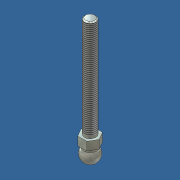
# Autodesk Inventor part: 21.1846 THREADED STUD 10mm
Saved by Autodesk Inventor 2016 (Build 200138000, 138)
## iProperties
Created: 2007-03-28
Part Number: 21.1846 THREADED STUD 10mm
Document SubType Name: Modeling
Designer: Andy Moles
Material: Steel
Mass: 80.0158 g
Surface Area: 40.5758 cm^2
Volume: 10.1931 cm^3
Density: 7.85 g/cm^3
Appearance: Zinc
Author: Andy Moles
Autodesk Inventor part; units mm, degrees
ref_plane "YZ Plane" through (0, 0, 0) normal (1, 0, 0) x (0, 1, 0)
ref_plane "XZ Plane" through (0, 0, 0) normal (0, 1, 0) x (-1, 0, 0)
ref_plane "XY Plane" through (0, 0, 0) normal (0, 0, 1) x (1, 0, 0)
sketch "Sketch1" plane through (0, 0, 0) normal (0, 0, 1) x (1, 0, 0)
  arc A0 (0, -7.5) -> (0, 7.5) centre (0, 0) ccw
  line L0 (0, -7.5) -> (0, 7.5)
  dimension "d5" = 15
  constraints: 2 end point, 2 point on circle, 1 centre point, 1 coincident, 1 midpoint, 1 vertical
  measures "d5" distance of L0.start L0.end
revolve "Revolution1" add sketch "Sketch1" angle 360 about axis through (0, -7.5, 0) along (0, 1, 0)
sketch "Sketch2" plane through (0, 0, 0) normal (0, 0, 1) x (1, 0, 0)
  circle A0 centre (0, 0) radius 6
  dimension "d2" = 12
  constraints: 1 centre point, 1 coincident
  measures "d2" diameter of A0
extrude "Extrusion1" add sketch "Sketch2" along normal blind 7
sketch "Sketch3" plane through (0, 0, 7) normal (0, 0, 1) x (1, 0, 0)
  circle A0 centre (0, 0) radius 6 projected
  line L0 (-4.0415, 7) -> (4.0415, 7)
  line L1 (4.0415, 7) -> (8.0829, 0)
  line L2 (8.0829, 0) -> (4.0415, -7)
  line L3 (4.0415, -7) -> (-4.0415, -7)
  line L4 (-4.0415, -7) -> (-8.0829, 0)
  line L5 (-8.0829, 0) -> (-4.0415, 7)
  point P0 (0, -7)
  dimension "d6" = 120
  dimension "d7" = 120
  dimension "d8" = 14
  constraints: 12 end point, 5 equal length, 1 horizontal, 1 horizontal alignment, 1 midpoint, 1 parallel, 1 vertical alignment
  measures "d6" angle of L5 L4
  measures "d7" angle of L0 L5
  measures "d8" distance between parallel lines of L3 L0
extrude "Extrusion2" add sketch "Sketch3" along normal blind 7.5 contours A0 | L0 L1 L2 L3 L4 L5
sketch "Sketch4" plane through (0, 0, 14.5) normal (0, 0, 1) x (1, 0, 0)
  circle A0 centre (0, 0) radius 5
  point P0 (0, 0)
  dimension "d11" = 10
  constraints: 1 centre point, 1 coincident
  measures "d11" diameter of A0
extrude "Extrusion3" add sketch "Sketch4" along normal blind 90
thread "Thread1" size "M10x1.5" class "6g" standard "ANSI Metric M Profile" length 88 offset 2
chamfer "Chamfer1" distance 1 angle 45 1 edges at (-5, 0, 104.5)
body "Solid1"
